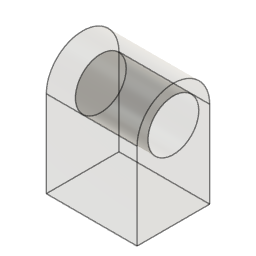
_End Mount for Smooth Rod (Autodesk Fusion 360 design; units mm, degrees)
part number: 2025-05-23-20-35-38-369
Autodesk Fusion 360 part; units mm, degrees
sketch "Sketch1" plane through (0, 0, 0) normal (1, 0, 0) x (0, 1, 0)
  line L0 (0, 0) -> (12, 0)
  line L1 (12, 0) -> (12, 14.3)
  line L2 (12, 14.3) -> (0, 14.3)
  line L3 (0, 14.3) -> (0, 0)
  circle A0 centre (6, 14.3) radius 6
  dimension "d1" = 12
  dimension "d2" = 14.3
  constraint horizontal L0
  constraint vertical L1
  constraint horizontal L2
  constraint vertical L3
  constraint coincident L0.start L3.end
  constraint midpoint L2 A0.centre
  constraint coincident L1.end A0
  measures "d1" distance of L0.start L0.end
  measures "d2" distance of L0.start L2.end
extrude "Extrude1" add sketch "Sketch1" along normal blind 15
hole "Hole1" at (15, 6, 14.3) direction (-1, 0, 0) diameter 8.4 depth 12 tip angle 180
